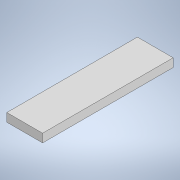
# Autodesk Inventor part: VerstaerkungHintenLinks
Saved by Autodesk Inventor 2020.3 (Build 243373010, 373A)
## iProperties
Created: 2021-02-13
Part Number: VerstaerkungHintenLinks
Material: Generisch
Document SubType Name: Modeling
Designer: Stefan
Density: 1 g/cm^3
Appearance: Vorgabe
Author: Stefan
Autodesk Inventor part; units mm, degrees
ref_plane "YZ Plane" through (0, 0, 0) normal (1, 0, 0) x (0, 1, 0)
ref_plane "XZ Plane" through (0, 0, 0) normal (0, 1, 0) x (-1, 0, 0)
ref_plane "XY Plane" through (0, 0, 0) normal (0, 0, 1) x (1, 0, 0)
sketch "Skizze1" plane through (0, 0, 0) normal (0, 1, 0) x (-1, 0, 0)
  line L0 (100.9437, 169.5604) -> (-41.0563, 169.5604)
  line L1 (-41.0563, 169.5604) -> (-41.0563, -140.4396)
  line L2 (-41.0563, -140.4396) -> (100.9437, -140.4396)
  line L3 (100.9437, -140.4396) -> (100.9437, 169.5604)
  point P0 (0, 0)
  dimension "d0" = 142
  dimension "d1" = 310
  constraints: 8 end point, 2 parallel, 1 horizontal, 1 perpendicular, 1 other
  measures "d0" distance of L1.end L2.end
  measures "d1" distance of L0.end L1.end
extrude "Extrusion1" add sketch "Skizze1" along normal blind 20
sketch "Skizze3" plane through (0, 20, 0) normal (0, 1, 0) x (1, 0, 0)
  line L0 (41.0563, -169.5604) -> (41.0563, 140.4396) projected
  line L1 (-100.9437, -169.5604) -> (41.0563, -169.5604) projected
  line L2 (41.0563, 140.4396) -> (-15.9437, 140.4396)
  line L3 (-15.9437, 140.4396) -> (-15.9437, -169.5604)
  line L4 (-15.9437, -169.5604) -> (41.0563, -169.5604)
  line L5 (41.0563, -169.5604) -> (41.0563, 140.4396)
  line L6 (-100.9437, 140.4396) -> (-100.9437, -169.5604) projected
  point P0 (0, 0)
  dimension "d66" = 85
  constraints: 8 end point, 2 parallel, 1 horizontal, 1 perpendicular, 1 point on line
  measures "d66" distance between parallel lines of L6 L3
extrude "Extrusion3" cut sketch "Skizze3" against normal through all
